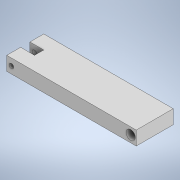
# Autodesk Inventor part: Ramp Base
Saved by Autodesk Inventor 2020 (Build 240168000, 168)
## iProperties
Created: 2021-01-30
Part Number: Ramp Base
Material: Generic
Document SubType Name: Modeling
Designer: magda
Density: 1 g/cm^3
Appearance: Default
Author: magda
Autodesk Inventor part; units mm, degrees
ref_plane "YZ Plane" through (0, 0, 0) normal (1, 0, 0) x (0, 1, 0)
ref_plane "XZ Plane" through (0, 0, 0) normal (0, 1, 0) x (-1, 0, 0)
ref_plane "XY Plane" through (0, 0, 0) normal (0, 0, 1) x (1, 0, 0)
sketch "Sketch1" plane through (0, 0, 0) normal (0, 0, 1) x (1, 0, 0)
  line L0 (-33.8048, 23.6808) -> (143.9952, 23.6808)
  line L1 (143.9952, 23.6808) -> (143.9952, 4.6308)
  line L2 (143.9952, 4.6308) -> (-33.8048, 4.6308)
  line L3 (-33.8048, 4.6308) -> (-33.8048, 23.6808)
  point P0 (0, 0)
  dimension "d0" = 177.8
  dimension "d1" = 19.05
  constraints: 8 end point, 2 parallel, 1 horizontal, 1 perpendicular
  measures "d0" distance of L1.end L2.end
  measures "d1" distance between parallel lines of L0 L2
extrude "Extrusion1" add sketch "Sketch1" along normal blind 50.8
sketch "Sketch2" plane through (0, 0, 50.8) normal (0, 0, 1) x (1, 0, 0)
  circle A0 centre (136.3752, 14.1558) radius 6.35
  line L0 (143.9952, 4.6308) -> (143.9952, 23.6808) projected
  line L1 (-33.8048, 4.6308) -> (143.9952, 4.6308) projected
  point P0 (0, 0)
  dimension "d4" = 12.7
  dimension "d5" = 7.62
  dimension "d6" = 9.525
  constraints: 1 centre point
  measures "d4" diameter of A0
  measures "d5" distance from line of L0 A0.centre
  measures "d6" distance from line of L1 A0.centre
extrude "Extrusion2" cut sketch "Sketch2" against normal blind 50.8
sketch "Sketch3" plane through (-33.8048, 23.6808, 0) normal (0, 1, 0) x (1, 0, 0)
  line L0 (0, 0) -> (0, -50.8) projected
  line L1 (0, -31.75) -> (19.05, -31.75)
  line L2 (19.05, -31.75) -> (19.05, -19.05)
  line L3 (19.05, -19.05) -> (0, -19.05)
  line L4 (0, -19.05) -> (0, -31.75)
  line L5 (177.8, 0) -> (0, 0) projected
  point P0 (33.8048, 0)
  point P1 (0, -19.05)
  dimension "d9" = 19.05
  dimension "d10" = 12.7
  dimension "d11" = 19.05
  constraints: 8 end point, 2 parallel, 1 horizontal, 1 perpendicular, 1 point on line
  measures "d9" distance of L3.end L2.end
  measures "d10" distance of L1.end L2.end
  measures "d11" distance between parallel lines of L5 L3
extrude "Extrusion3" cut sketch "Sketch3" against normal blind 50.8
sketch "Sketch4" plane through (-33.8048, 23.6808, 19.05) normal (0, 0, 1) x (1, 0, 0)
  circle A0 centre (6.35, -9.525) radius 3.175
  line L0 (19.05, 0) -> (19.05, -19.05) projected
  line L1 (0, -19.05) -> (177.8, -19.05) projected
  point P0 (33.8048, -23.6808)
  dimension "d14" = 6.35
  dimension "d15" = 12.7
  dimension "d16" = 9.525
  constraints: 1 centre point
  measures "d14" diameter of A0
  measures "d15" distance from line of L0 A0.centre
  measures "d16" distance from line of L1 A0.centre
extrude "Extrusion4" cut sketch "Sketch4" along normal mid plane 127
body "Solid1"
